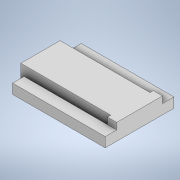
# Autodesk Inventor part: chaimber-bolt
Saved by Autodesk Inventor 2021 (Build 250183000, 183)
## iProperties
Created: 2024-03-14
Part Number: chaimber-bolt
Material: Generic
Document SubType Name: Modeling
Designer: 22hamfri
Density: 1 g/cm^3
Appearance: Default
Author: 22hamfri
Autodesk Inventor part; units mm, degrees
ref_plane "YZ Plane" through (0, 0, 0) normal (1, 0, 0) x (0, 1, 0)
ref_plane "XZ Plane" through (0, 0, 0) normal (0, 1, 0) x (-1, 0, 0)
ref_plane "XY Plane" through (0, 0, 0) normal (0, 0, 1) x (1, 0, 0)
sketch "Sketch1" plane through (0, 0, 0) normal (0, 1, 0) x (-1, 0, 0)
  line L0 (-24.5, 12) -> (24.5, 12)
  line L1 (24.5, 12) -> (24.5, -12)
  line L2 (24.5, -12) -> (-24.5, -12)
  line L3 (-24.5, -12) -> (-24.5, 12)
  line L4 (-24.5, 12) -> (24.5, -12) construction
  line L5 (24.5, 12) -> (-24.5, -12) construction
  line L6 (24.5, 12) -> (24.5, -12)
  line L7 (24.5, -12) -> (28.5, -12)
  line L8 (28.5, -12) -> (28.5, 12)
  line L9 (28.5, 12) -> (24.5, 12)
  line L10 (-24.5, -12) -> (-24.5, -14)
  line L11 (-24.5, -14) -> (24.5, -14)
  line L12 (24.5, -14) -> (24.5, -21)
  line L13 (24.5, -21) -> (-32.1, -21)
  line L14 (-32.1, -21) -> (-32.1, 0)
  line L15 (28.5, 0) -> (-32.1, 0)
  line L16 (-24.5, -12) -> (-32.1, -12)
  line L17 (-24.5, -14) -> (-32.1, -14)
  line L18 (24.5, 12) -> (-24.5, 12)
  line L19 (24.5, 12) -> (28.5, 12)
  line L20 (-24.5, 12) -> (-24.5, 14)
  line L21 (-24.5, 14) -> (24.5, 14)
  line L22 (24.5, 14) -> (24.5, 21)
  line L23 (24.5, 21) -> (-32.1, 21)
  line L24 (-32.1, 21) -> (-32.1, 0)
  line L25 (-24.5, 12) -> (-32.1, 12)
  line L26 (-24.5, 14) -> (-32.1, 14)
  line L27 (-26.5, -12) -> (-26.5, -14)
  line L28 (-26.5, 14) -> (-26.5, 12)
  point P0 (0, 0)
  dimension "d0" = 24
  dimension "d1" = 49
  dimension "d2" = 7
  dimension "d3" = 2
  dimension "d4" = 7.6
  dimension "d5" = 4
  dimension "d12" = 2
  constraints: 58 end point, 8 perpendicular, 8 point on line, 6 symmetric about line, 5 equal length, 3 midpoint, 2 collinear, 2 horizontal, 1 vertical
  measures "d0" distance between parallel lines of L2 L0
  measures "d1" distance between parallel lines of L3 L1
  measures "d2" distance between parallel lines of L13 L11
  measures "d3" distance between parallel lines of L11 L7
  measures "d4" distance between parallel lines of L3 L14
  measures "d5" distance between parallel lines of L8 L1
  measures "d12" distance between parallel lines of L3 L27
extrude "Extrusion1" add sketch "Sketch1" along normal blind 10 contours L0 L1 L15 L3 | L3 L15 L24 L25 | L9 L8 L15 L1 | L15 L1 L2 L3 | L3 L16 L14 L15 | L25 L24 L26 L28 | L15 L8 L7 L1 | L27 L17 L14 L16
extrude "Extrusion2" add sketch "Sketch1" along normal blind 6 contours L26 L24 L23 L22 L21 | L11 L12 L13 L14 L17
body "Solid1"
